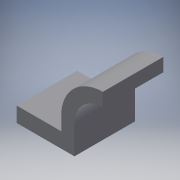
# Autodesk Inventor part: solenoid_mount
Saved by Autodesk Inventor 2016 (Build 200138000, 138)
## iProperties
Created: 2016-01-27
Part Number: solenoid_mount
Material: Generic
Document SubType Name: Modeling
Designer: seve
Density: 1 g/cm^3
Appearance: Default
Author: seve
Autodesk Inventor part; units mm, degrees
ref_plane "YZ Plane" through (0, 0, 0) normal (1, 0, 0) x (0, 1, 0)
ref_plane "XZ Plane" through (0, 0, 0) normal (0, 1, 0) x (-1, 0, 0)
ref_plane "XY Plane" through (0, 0, 0) normal (0, 0, 1) x (1, 0, 0)
sketch "Sketch1" plane through (0, 0, 0) normal (0, 0, 1) x (1, 0, 0)
  circle A0 centre (0, 0) radius 5.9643 projected
  line L0 (-5.9643, -5.9643) -> (-5.9643, 0)
  line L1 (-5.9643, -5.9643) -> (-18.0863, -5.9643)
  line L2 (-18.0863, -5.9643) -> (-18.0863, -2.7893)
  line L3 (-18.0863, -2.7893) -> (-8.7535, -2.7893)
  line L4 (-8.7535, -2.7893) -> (-8.7535, 0)
  line L5 (-6.4071, -5.9643) -> (-18.0863, -5.9643)
  line L6 (-8.7535, -2.7893) -> (-8.7535, 0)
  arc A1 (0, 5.9643) -> (-5.9643, 0) centre (0, 0) ccw
  line L7 (-5.9643, -5.9643) -> (-6.4071, -5.9643)
  line L8 (0, 5.9643) -> (0, 8.7535)
  arc A2 (0, 8.7535) -> (-8.7535, 0) centre (0, 0) ccw
  dimension "d0" = 3.175
  constraints: 18 end point, 4 point on circle, 3 perpendicular, 2 centre point, 2 coincident, 2 vertical, 1 collinear, 1 horizontal, 1 horizontal alignment, 1 point on line, 1 tangent, 2 other
  measures "d0" distance of L1.end L2.end
extrude "Extrusion1" add sketch "Sketch1" along normal blind 12.7 contours A0 L0 L1 L2 L3 L4 A2 L8
sketch "Sketch2" plane through (-18.0863, -2.7893, 0) normal (0, 1, 0) x (1, 0, 0)
  point P0 (18.0863, 0)
  point P1 (4.3814, -3.415)
  point P2 (4.3814, -8.5375)
hole "Hole1" at (-13.7049, -2.7893, 3.415) at (-13.7049, -2.7893, 8.5375) direction (0, -1, 0) diameter 1.5875 end through all
body "Solid1"
